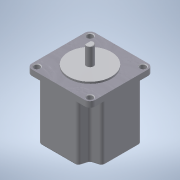
# Autodesk Inventor part: nema 23 stepper
Saved by Autodesk Inventor 2020 (Build 240168000, 168)
## iProperties
Created: 2013-09-07
Part Number: nema 23 stepper
Document SubType Name: Modeling
Designer: Ja
Density: 7.85 g/cm^3
Material: Steel, High Strength, Low Alloy
Appearance: White
Author: Ja
Autodesk Inventor part; units mm, degrees
ref_plane "YZ Plane" through (0, 0, 0) normal (1, 0, 0) x (0, 1, 0)
ref_plane "XZ Plane" through (0, 0, 0) normal (0, 1, 0) x (-1, 0, 0)
ref_plane "XY Plane" through (0, 0, 0) normal (0, 0, 1) x (1, 0, 0)
sketch "Náčrt1" plane through (0, 0, 0) normal (0, 0, 1) x (1, 0, 0)
  line L0 (0, 0) -> (-28.2, 0)
  line L1 (-28.2, 0) -> (-28.2, -28.2)
  line L2 (-28.2, -28.2) -> (0, -28.2)
  line L3 (0, -28.2) -> (28.2, -28.2)
  line L4 (28.2, -28.2) -> (28.2, 28.2)
  line L5 (28.2, 28.2) -> (-28.2, 28.2)
  line L6 (-28.2, 28.2) -> (-28.2, 0)
  dimension "d0" = 28.2
  dimension "d1" = 28.2
  dimension "d2" = 28.2
  dimension "d3" = 56.4
  constraints: 14 end point, 4 parallel, 1 collinear, 1 horizontal, 1 perpendicular
  measures "d0" distance of L0.start L0.end
  measures "d1" distance of L0.end L1.end
  measures "d2" distance of L2.end L3.end
  measures "d3" distance of L3.end L4.end
extrude "Vysunutí1" add sketch "Náčrt1" along normal blind 54
sketch "Náčrt2" plane through (0, 0, 0) normal (0, 0, -1) x (-1, 0, 0)
  line L0 (28.2, 28.2) -> (28.2, -28.2) projected
  line L1 (-28.2, 28.2) -> (28.2, 28.2) projected
  line L2 (-28.2, -28.2) -> (-28.2, 28.2) projected
  line L3 (28.2, -28.2) -> (-28.2, -28.2) projected
  line L4 (28.2, 0) -> (28.2, -17.25)
  line L5 (17.25, -28.2) -> (-17.25, -28.2)
  line L6 (-17.25, -28.2) -> (-28.2, -17.25)
  line L7 (-28.2, -17.25) -> (-28.2, 17.25)
  line L8 (-28.2, 17.25) -> (-17.25, 28.2)
  line L9 (17.25, 28.2) -> (28.2, 17.25)
  line L10 (28.2, 17.25) -> (28.2, 0)
  line L11 (28.2, -28.2) -> (19.7, -28.2)
  line L12 (19.7, -28.2) -> (19.7, -19.7)
  line L13 (19.7, -19.7) -> (28.2, -19.7)
  line L14 (28.2, -19.7) -> (28.2, -28.2)
  line L15 (-28.2, -28.2) -> (-19.7, -28.2)
  line L16 (-19.7, -28.2) -> (-19.7, -19.7)
  line L17 (-19.7, -19.7) -> (-28.2, -19.7)
  line L18 (-28.2, -19.7) -> (-28.2, -28.2)
  line L19 (-28.2, 28.2) -> (-19.7, 28.2)
  line L20 (-19.7, 28.2) -> (-19.7, 19.7)
  line L21 (-19.7, 19.7) -> (-28.2, 19.7)
  line L22 (-28.2, 19.7) -> (-28.2, 28.2)
  line L23 (28.2, 28.2) -> (19.7, 28.2)
  line L24 (19.7, 28.2) -> (19.7, 19.7)
  line L25 (19.7, 19.7) -> (28.2, 19.7)
  line L26 (28.2, 19.7) -> (28.2, 28.2)
  line L27 (28.2, 17.25) -> (19.7, 19.7)
  line L28 (17.25, 28.2) -> (19.7, 19.7)
  line L29 (-17.25, 28.2) -> (-19.7, 19.7)
  line L30 (-28.2, 17.25) -> (-19.7, 19.7)
  line L31 (-28.2, -17.25) -> (-19.7, -19.7)
  line L32 (-19.7, -19.7) -> (-17.25, -28.2)
  line L33 (17.25, -28.2) -> (19.7, -19.7)
  line L34 (19.7, -19.7) -> (28.2, -17.25)
  line L35 (28.2, -17.25) -> (25.75, -19.7)
  line L36 (19.7, -25.75) -> (17.25, -28.2)
  point P0 (0, 0)
  dimension "d6" = 17.25
  dimension "d8" = 34.5
  dimension "d9" = 34.5
  dimension "d10" = 8.5
  dimension "d11" = 8.5
  dimension "d12" = 8.5
  dimension "d13" = 8.5
  dimension "d14" = 8.5
  constraints: 66 end point, 11 perpendicular, 10 point on line, 9 parallel, 4 horizontal, 1 midpoint
  measures "d6" distance of L4.start L4.end
  measures "d8" distance of L5.start L5.end
  measures "d9" distance of L6.end L7.end
  measures "d10" distance of L12.end L13.end
  measures "d11" distance of L11.end L12.end
  measures "d12" distance of L17.end L16.end
  measures "d13" distance of L16.end L15.end
  measures "d14" distance of L19.end L20.end
extrude "Vysunutí2" add sketch "Náčrt2" along normal blind 49 contours L0 L34 L33 L3 L32 L31 L2 L30 L29 L1 L28 L27
sketch "Náčrt3" plane through (0, 0, 54) normal (0, 0, 1) x (1, 0, 0)
  line L0 (-28.2, -28.2) -> (-28.2, 28.2) projected
  line L1 (28.2, -28.2) -> (-28.2, -28.2) projected
  line L2 (28.2, -28.2) -> (-28.2, -28.2)
  line L3 (-28.2, -28.2) -> (-28.2, 28.2)
  line L4 (-28.2, 28.2) -> (28.2, 28.2)
  line L5 (28.2, 28.2) -> (28.2, -28.2)
  point P0 (0, 0)
  constraints: 8 end point, 2 parallel, 1 horizontal, 1 perpendicular
extrude "Vysunutí3" cut sketch "Náčrt3" against normal blind 49
fillet "Zaoblení1" radius 3 12 edges at (-17.25, -28.2, -24.5) (-19.7, -19.7, -24.5) (-28.2, -17.25, -24.5) (17.25, -28.2, -24.5) (19.7, -19.7, -24.5) (28.2, -17.25, -24.5) (28.2, 17.25, -24.5) (19.7, 19.7, -24.5) (17.25, 28.2, -24.5) (-17.25, 28.2, -24.5) (-19.7, 19.7, -24.5) (-28.2, 17.25, -24.5)
fillet "Zaoblení2" radius 4.6 4 edges at (28.2, 28.2, 2.5) (28.2, -28.2, 2.5) (-28.2, -28.2, 2.5) (-28.2, 28.2, 2.5)
sketch "Náčrt4" plane through (0, 0, 5) normal (0, 0, 1) x (1, 0, 0)
  circle A0 centre (0, 0) radius 19.05
  dimension "d21" = 38.1
  constraints: 1 centre point, 1 coincident
  measures "d21" diameter of A0
extrude "Vysunutí4" add sketch "Náčrt4" along normal blind 1.6
sketch "Náčrt5" plane through (0, 0, 6.6) normal (0, 0, 1) x (1, 0, 0)
  circle A0 centre (0, 0) radius 19.05 projected
  circle A1 centre (0, 0) radius 3.175
  dimension "d24" = 6.35
  constraints: 1 centre point, 1 coincident
  measures "d24" diameter of A1
extrude "Vysunutí5" add sketch "Náčrt5" along normal blind 16 contours A1
sketch "Náčrt6" plane through (0, 0, 5) normal (0, 0, 1) x (1, 0, 0)
  arc A0 (-23.6, 28.2) -> (-28.2, 23.6) centre (-23.6, 23.6) ccw projected
hole "Díra1" at (-23.6, 23.6, 5) direction (0, 0, -1) diameter 5.2 end through all
sketch "Náčrt7" plane through (0, 0, 5) normal (0, 0, 1) x (1, 0, 0)
  arc A0 (28.2, 23.6) -> (23.6, 28.2) centre (23.6, 23.6) ccw projected
hole "Díra2" at (23.6, 23.6, 5) direction (0, 0, -1) diameter 5.2 end through all
sketch "Náčrt8" plane through (0, 0, 5) normal (0, 0, 1) x (1, 0, 0)
  arc A0 (23.6, -28.2) -> (28.2, -23.6) centre (23.6, -23.6) ccw projected
hole "Díra3" at (23.6, -23.6, 5) direction (0, 0, -1) diameter 5.2 end through all
sketch "Náčrt9" plane through (0, 0, 5) normal (0, 0, 1) x (1, 0, 0)
  arc A0 (-28.2, -23.6) -> (-23.6, -28.2) centre (-23.6, -23.6) ccw projected
hole "Díra4" at (-23.6, -23.6, 5) direction (0, 0, -1) diameter 5.2 end through all
sketch "Náčrt10" plane through (0, 0, -49) normal (0, 0, -1) x (-1, 0, 0)
  point P0 (0, 0)
hole "Díra5" at (0, 0, -49) direction (0, 0, 1) diameter 8.5 depth 5 countersink diameter 9 countersink angle 90
sketch "Náčrt15" plane through (0, 0, 22.6) normal (0, 0, 1) x (1, 0, 0)
  circle A0 centre (0, 0) radius 3.175 projected
  line L0 (-1.9907, -2.4734) -> (-1.9907, 2.4734)
  constraints: 2 end point, 2 point on circle, 1 vertical
extrude "Vysunutí10" cut sketch "Náčrt15" against normal blind 10 contours L0 A0 picked at (-2.3855, 0)
chamfer "Zkosení1" distance 0.4 angle 45 3 edges at (-1.9907, 0, 22.6) (1.3712, -2.8637, 22.6) (1.3712, 2.8637, 22.6)
chamfer "Zkosení2" distance 0.5 angle 45 8 edges at (-23.6, 26.2, 5) (23.6, 26.2, 5) (23.6, -21, 5) (-23.6, -21, 5) (-23.6, -21, 0) (23.6, -21, 0) (23.6, 26.2, 0) (-23.6, 26.2, 0)
fillet "Zaoblení3" radius 0.8 24 edges at (0, 28.2, -49) (-16.7964, 27.5971, -49) (-18.5581, 23.6618, -49) (-20.0023, 20.0023, -49) (-23.6618, 18.5581, -49) (-27.5971, 16.7964, -49) (-28.2, 0, -49) (-27.5971, -16.7964, -49) (-23.6618, -18.5581, -49) (-20.0023, -20.0023, -49) (-18.5581, -23.6618, -49) (-16.7964, -27.5971, -49) (0, -28.2, -49) (16.7964, -27.5971, -49) (18.5581, -23.6618, -49) (20.0023, -20.0023, -49) (23.6618, -18.5581, -49) (27.5971, -16.7964, -49) (28.2, 0, -49) (27.5971, 16.7964, -49) (23.6618, 18.5581, -49) (20.0023, 20.0023, -49) (18.5581, 23.6618, -49) (16.7964, 27.5971, -49)
